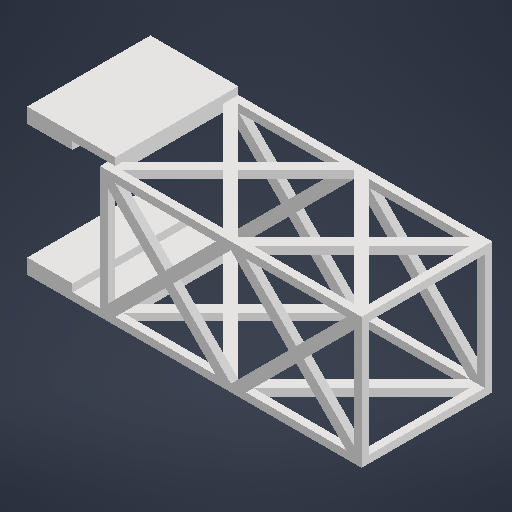
# Autodesk Inventor part: 足フレーム
Saved by Autodesk Inventor 2026 (Build 300175000, 175)
## iProperties
Created: 2025-10-26
Part Number: 足フレーム
Material: 一般
Document SubType Name: Modeling
Designer: masak
Density: 1 g/cm^3
Appearance: 既定
Author: masak
Autodesk Inventor part; units mm, degrees
ref_plane "YZ Plane" through (0, 0, 0) normal (1, 0, 0) x (0, 1, 0)
ref_plane "XZ Plane" through (0, 0, 0) normal (0, 1, 0) x (-1, 0, 0)
ref_plane "XY Plane" through (0, 0, 0) normal (0, 0, 1) x (1, 0, 0)
sketch "スケッチ1" plane through (0, 0, 0) normal (0, 0, 1) x (1, 0, 0)
  line L0 (-11.5, 13) -> (-11.5, -13) projected
  line L1 (11.5, 13) -> (-11.5, 13) projected
  line L2 (11.5, -13) -> (11.5, 13) projected
  line L3 (-11.5, -13) -> (11.5, -13) projected
  line L4 (11.5, 13) -> (63.5, 13)
  line L5 (63.5, 13) -> (63.5, -13)
  line L6 (63.5, -13) -> (11.5, -13)
  line L7 (11.5, -13) -> (11.5, 13)
  line L8 (37.5, 13) -> (37.5, -13)
  line L9 (11.5, 13) -> (37.5, -13)
  line L10 (37.5, 13) -> (11.5, -13)
  line L11 (63.5, 13) -> (37.5, -13)
  line L12 (37.5, 13) -> (63.5, -13)
  line L13 (13, -11.5) -> (62, -11.5)
  line L14 (62, 11.5) -> (13, 11.5)
  line L15 (13, -11.5) -> (13, 11.5)
  line L16 (62, -11.5) -> (62, 11.5)
  line L17 (13, -13) -> (37.5, 11.5)
  line L18 (11.5, -11.5) -> (36, 13)
  line L19 (37.5, -11.5) -> (14.5, 11.5)
  line L20 (13, 10) -> (36, -13)
  line L21 (37.5, -11.5) -> (60.5, 11.5)
  line L22 (62, 10) -> (39, -13)
  line L23 (38.0069, 10.9931) -> (60.5, -11.5)
  line L24 (62, -10) -> (39, 13)
  line L25 (37.5, 11.5) -> (60.5, -11.5)
  point P0 (0, 0)
  point P1 (49, 0)
  point P2 (26, 0)
  point P3 (13, -10)
  point P4 (23, 0)
  point P5 (34.5, 11.5)
  point P6 (24.5, 1.5)
  point P7 (14.5, -11.5)
  point P8 (24.5, -1.5)
  point P9 (34.5, -11.5)
  point P10 (40.5, -11.5)
  point P11 (50.5, -1.5)
  point P12 (52, 0)
  point P13 (40.5, 11.5)
  point P14 (50.5, 1.5)
  dimension "d0" = 52
  dimension "d1" = 26
  dimension "d2" = 1.5
  constraints: 44 end point, 19 point on line, 7 perpendicular, 6 parallel, 4 midpoint, 2 horizontal
  measures "d0" distance of L1.start L4.end
  measures "d1" distance of L4.end L5.end
  measures "d2" distance from line of L6 L13.start
extrude "押し出し1" add sketch "スケッチ1" against normal blind 1.5 contours L9 L15 L18 L2 | L4 L18 L14 L9 | L10 L13 L17 L6 | L2 L18 L15 L10 | L4 L10 L14 L18 | L14 L19 L18 L9 | L9 L18 L20 L15 | L17 L13 L20 L6 | L15 L18 L20 L10 | L10 L20 L17 L13 | L12 L14 L8 | L8 L14 L10 | L4 L24 L14 L12 | L14 L10 L19 L18 | L18 L19 L10 L9 | L9 L10 L20 L18 | L20 L13 L9 L6 | L10 L9 L17 L20 | L4 L11 L14 L24 | L17 L19 L10 L14 | L14 L12 L21 L23 L25 | L14 L24 L21 L12 | L10 L19 L17 L9 | L11 L13 L22 L6 | L9 L13 L8 | L8 L13 L11 | L20 L17 L9 L13 | L5 L12 L16 L11 | L21 L23 L11 L13 | L13 L9 L17 L19 | L21 L24 L11 L12 | L12 L11 L23 L21 | L22 L13 L12 L6 | L11 L23 L22 L13 | L16 L22 L24 L11 | L11 L24 L21 L14 | L12 L22 L23 L11 | L11 L24 L22 L12 | L13 L23 L22 L12 | L12 L22 L24 L16
sketch "スケッチ5" plane through (11.5, 13, 0) normal (0, 1, 0) x (1, 0, 0)
  line L0 (-7, 32) -> (0, 32) projected
  line L1 (0, 32) -> (0, 0) projected
  line L2 (0, 0) -> (-23, 0) projected
  line L3 (52, 0) -> (0, 0) projected
  line L4 (52, 0) -> (52, 26)
  line L5 (52, 26) -> (0, 26)
  line L6 (1.5, 26) -> (1.5, 0)
  line L7 (0, 24.5) -> (52, 24.5)
  line L8 (50.5, 26) -> (50.5, 0)
  line L9 (0, 1.5) -> (52, 1.5) projected
  line L10 (26, 1.5) -> (26, 26)
  line L11 (0, 26) -> (26, 0)
  line L12 (52, 26) -> (26, 0)
  line L13 (1.5, 26) -> (26, 1.5)
  line L14 (26, 1.5) -> (50.5, 26)
  line L15 (52, 24.5) -> (27.5, 0)
  line L16 (24.5, 0) -> (0, 24.5)
  line L17 (0, 0) -> (26, 26)
  line L18 (26, 26) -> (52, 0)
  line L19 (52, 1.5) -> (27.5, 26)
  line L20 (26, 24.5) -> (50.5, 0)
  line L21 (26, 24.5) -> (1.5, 0)
  line L22 (0, 1.5) -> (24.5, 26)
  point P0 (-11.5, 0)
  point P1 (49, 1.5)
  point P2 (29, 1.5)
  point P3 (39, 11.5)
  point P4 (14.5, 13)
  point P5 (37.5, 13)
  point P6 (3, 1.5)
  point P7 (13, 11.5)
  point P8 (23, 1.5)
  point P9 (50.5, 3)
  point P10 (40.5, 13)
  point P11 (50.5, 23)
  point P12 (29, 24.5)
  point P13 (49, 24.5)
  point P14 (39, 14.5)
  point P15 (1.5, 3)
  point P16 (1.5, 23)
  point P17 (11.5, 13)
  point P18 (3, 24.5)
  point P19 (23, 24.5)
  point P20 (13, 14.5)
  dimension "d7" = 26
  dimension "d8" = 1.5
  dimension "d9" = 1.5
  dimension "d10" = 1.5
  constraints: 34 end point, 13 point on line, 5 perpendicular, 3 midpoint, 2 vertical, 1 parallel, 10 other
  measures "d7" distance of L3.start L4.end
  measures "d8" distance of L6.start L11.start
  measures "d9" distance of L7.end L4.end
  measures "d10" distance of L4.end L8.start
extrude "押し出し2" add sketch "スケッチ5" against normal blind 1.5 contours L11 L7 L1 | L5 L6 L11 | L16 L6 L22 L1 | L7 L6 L16 | L13 L7 L6 | L5 L22 L7 L13 | L11 L22 L16 L6 | L7 L13 L22 L11 | L9 L17 L1 | L22 L6 L9 | L5 L17 L7 L22 | L22 L13 L17 L11 | L11 L17 L16 L22 | L17 L6 L3 | L9 L21 L6 | L17 L16 L21 L9 | L6 L22 L16 L17 | L18 L7 L10 | L10 L7 L17 | L5 L19 L7 L18 | L7 L17 L13 L22 | L17 L13 L21 L11 | L11 L21 L16 L17 | L21 L9 L16 L3 | L5 L14 L7 L19 | L21 L13 L17 L7 | L7 L18 L14 L20 | L7 L19 L14 L18 | L21 L13 L9 L11 | L11 L9 L16 L21 | L16 L9 L11 L3 | L5 L12 L8 | L8 L7 L14 | L9 L12 L11 | L14 L20 L12 L9 | L14 L18 L12 L20 | L14 L19 L12 L18 | L12 L9 L15 L3 | L4 L7 L12 | L12 L19 L14 L7 | L7 L15 L8 | L8 L15 L19 L12 | L12 L20 L15 L9 | L12 L18 L15 L20 | L12 L19 L15 L18 | L15 L9 L20 L3 | L4 L19 L8 L15 | L15 L18 L9 L20 | L15 L19 L8 L18 | L8 L18 L3 | L20 L9 L8 | L4 L18 L9 | L9 L8 L19
sketch "スケッチ6" plane through (11.5, -13, 0) normal (0, -1, 0) x (1, 0, 0)
  line L0 (1.5, -3) -> (11.5, -13) projected
  line L1 (13, -11.5) -> (3, -1.5) projected
  line L2 (52, -1.5) -> (0, -1.5) projected
  line L3 (0, 0) -> (52, 0) projected
  line L4 (0, -32) -> (0, 0) projected
  line L5 (1.5, -23) -> (1.5, -3) projected
  line L6 (11.5, -13) -> (1.5, -23) projected
  line L7 (3, -24.5) -> (13, -14.5) projected
  line L8 (23, -24.5) -> (3, -24.5) projected
  line L9 (0, -26) -> (52, -26) projected
  line L10 (13, -14.5) -> (23, -24.5) projected
  line L11 (26, -24.5) -> (14.5, -13) projected
  line L12 (14.5, -13) -> (26, -1.5) projected
  line L13 (23, -1.5) -> (13, -11.5) projected
  line L14 (39, -11.5) -> (29, -1.5) projected
  line L15 (26, -1.5) -> (37.5, -13) projected
  line L16 (29, -24.5) -> (39, -14.5) projected
  line L17 (37.5, -13) -> (26, -24.5) projected
  line L18 (49, -24.5) -> (29, -24.5) projected
  line L19 (39, -14.5) -> (49, -24.5) projected
  line L20 (50.5, -23) -> (40.5, -13) projected
  line L21 (50.5, -3) -> (50.5, -23) projected
  line L22 (52, -26) -> (52, -1.5) projected
  line L23 (40.5, -13) -> (50.5, -3) projected
  line L24 (49, -1.5) -> (39, -11.5) projected
  line L25 (52, 0) -> (52, -1.5) projected
  point P0 (-11.5, 0)
extrude "押し出し3" add sketch "スケッチ6" against normal blind 1.5 contours L13 L2 L14 L24 L22 L9 L4 L1 | L2 L4 L3 L25
sketch "スケッチ7" plane through (63.5, 13, -26) normal (0, 0, -1) x (-1, 0, 0)
  line L0 (50.5, -3) -> (50.5, -23) projected
  line L1 (40.5, -13) -> (50.5, -3) projected
  line L2 (49, -1.5) -> (39, -11.5) projected
  line L3 (52, -1.5) -> (0, -1.5) projected
  line L4 (39, -11.5) -> (29, -1.5) projected
  line L5 (26, -1.5) -> (37.5, -13) projected
  line L6 (37.5, -13) -> (26, -24.5) projected
  line L7 (29, -24.5) -> (39, -14.5) projected
  line L8 (39, -14.5) -> (49, -24.5) projected
  line L9 (0, -24.5) -> (52, -24.5) projected
  line L10 (52, 0) -> (52, -7) projected
  line L11 (52, -19) -> (52, -7) projected
  line L12 (52, -19) -> (52, -26) projected
  line L13 (52, -26) -> (0, -26) projected
  line L14 (0, 0) -> (52, 0) projected
  line L15 (14.5, -13) -> (26, -1.5) projected
  line L16 (26, -24.5) -> (14.5, -13) projected
  line L17 (13, -14.5) -> (23, -24.5) projected
  line L18 (3, -24.5) -> (13, -14.5) projected
  line L19 (11.5, -13) -> (1.5, -23) projected
  line L20 (1.5, -3) -> (11.5, -13) projected
  line L21 (13, -11.5) -> (3, -1.5) projected
  line L22 (23, -1.5) -> (13, -11.5) projected
  line L23 (1.5, -23) -> (1.5, -3) projected
  line L24 (0, -1.5) -> (0, -24.5) projected
  line L25 (0, 0) -> (0, -1.5) projected
  line L26 (0, -26) -> (0, -24.5) projected
  line L27 (50.5, -23) -> (40.5, -13) projected
  point P0 (63.5, -13)
extrude "押し出し4" add sketch "スケッチ7" against normal blind 1.5 contours L3 L10 L11 L12 L9 L8 L7 L6 L5 L4 L2 | L3 L25 L14 L10 | L15 L16 L9 L17 L18 L24 L3 L21 L22 | L12 L13 L26 L9
sketch "スケッチ8" plane through (0, 0, 0) normal (0, 0, 1) x (1, 0, 0)
  line L0 (11.5, 13) -> (-11.5, 13) projected
  line L1 (11.5, -13) -> (11.5, 13) projected
  line L2 (11.5, 13) -> (-11.5, 13) projected
  line L3 (-11.5, 13) -> (-11.5, -13) projected
  line L4 (-11.5, -13) -> (11.5, -13) projected
  circle A0 centre (0, 0) radius 5 projected
  line L5 (40.5, -11.5) -> (50.5, -1.5) projected
  line L6 (50.5, -1.5) -> (60.5, -11.5) projected
  line L7 (60.5, -11.5) -> (40.5, -11.5) projected
  line L8 (63.5, -13) -> (63.5, 13) projected
  line L9 (63.5, 13) -> (11.5, 13) projected
  line L10 (11.5, 13) -> (11.5, -13) projected
  line L11 (11.5, -13) -> (63.5, -13) projected
  line L12 (37.5, -11.5) -> (26, 0) projected
  line L13 (26, 0) -> (37.5, 11.5) projected
  line L14 (37.5, 11.5) -> (49, 0) projected
  line L15 (49, 0) -> (37.5, -11.5) projected
  line L16 (34.5, -11.5) -> (14.5, -11.5) projected
  line L17 (14.5, -11.5) -> (24.5, -1.5) projected
  line L18 (24.5, -1.5) -> (34.5, -11.5) projected
  line L19 (34.5, 11.5) -> (24.5, 1.5) projected
  line L20 (24.5, 1.5) -> (14.5, 11.5) projected
  line L21 (14.5, 11.5) -> (34.5, 11.5) projected
  line L22 (40.5, 11.5) -> (60.5, 11.5) projected
  line L23 (60.5, 11.5) -> (50.5, 1.5) projected
  line L24 (50.5, 1.5) -> (40.5, 11.5) projected
  line L25 (13, -10) -> (13, 10) projected
  line L26 (13, 10) -> (23, 0) projected
  line L27 (23, 0) -> (13, -10) projected
  line L28 (52, 0) -> (62, 10) projected
  line L29 (62, 10) -> (62, -10) projected
  line L30 (62, -10) -> (52, 0) projected
  line L31 (13, 10) -> (13, 14.5)
  line L32 (4.5, 13) -> (4.5, 11.5) projected
  line L33 (4.5, 11.5) -> (10, 11.5) projected
  line L34 (10, 11.5) -> (10, 6) projected
  line L35 (10, 6) -> (11.5, 6) projected
  line L36 (-4.5, 11.5) -> (-4.5, 13) projected
  line L37 (-10, 11.5) -> (-4.5, 11.5) projected
  line L38 (-10, 6) -> (-10, 11.5) projected
  line L39 (-11.5, 6) -> (-10, 6) projected
  line L40 (13, 14.5) -> (-4.5, 14.5)
  line L41 (-4.5, 14.5) -> (-4.5, 11.5)
  line L42 (-4.5, 11.5) -> (4.5, 11.5)
  line L43 (4.5, 13) -> (11.5, 13)
  line L44 (-4.5, -13) -> (-4.5, -11.5) projected
  line L45 (-4.5, -11.5) -> (-10, -11.5) projected
  line L46 (-10, -11.5) -> (-10, -6) projected
  line L47 (-10, -6) -> (-11.5, -6) projected
  line L48 (4.5, -11.5) -> (4.5, -13) projected
  line L49 (10, -11.5) -> (4.5, -11.5) projected
  line L50 (10, -6) -> (10, -11.5) projected
  line L51 (11.5, -6) -> (10, -6) projected
  line L52 (13, -13) -> (23, -13) projected
  line L53 (13, -13) -> (13, -14.5)
  line L54 (13, -14.5) -> (-4.5, -14.5)
  line L55 (-4.5, -14.5) -> (-4.5, -11.5)
  line L56 (-4.5, -11.5) -> (4.5, -11.5)
  line L57 (4.5, -13) -> (4.5, -11.5)
  line L58 (4.5, -13) -> (11.5, -13)
  point P0 (13, 12.25)
  point P1 (13, 13)
  dimension "d17" = 4.5
  dimension "d19" = 1.5
  constraints: 22 end point, 5 perpendicular, 2 collinear, 2 horizontal, 2 vertical, 1 midpoint, 1 other
  measures "d17" distance of L25.end L31.end
  measures "d19" distance of L52.start L53.end
extrude "押し出し5" add sketch "スケッチ8" against normal blind 24.5 from surface at -1.5 contours L0 L41 L40 L31 L9 | L32 L42 L36 L0 | L11 L53 L54 L55 L4 | L4 L44 L56 L48
